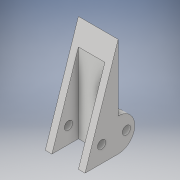
# Autodesk Inventor part: Scooop
Saved by Autodesk Inventor 2019 (Build 230136000, 136)
## iProperties
Created: 2019-05-08
Part Number: Scooop
Material: Generic
Document SubType Name: Modeling
Designer: codubois20
Density: 1 g/cm^3
Appearance: Default
Author: codubois20
Autodesk Inventor part; units mm, degrees
ref_plane "YZ Plane" through (0, 0, 0) normal (1, 0, 0) x (0, 1, 0)
ref_plane "XZ Plane" through (0, 0, 0) normal (0, 1, 0) x (-1, 0, 0)
ref_plane "XY Plane" through (0, 0, 0) normal (0, 0, 1) x (1, 0, 0)
sketch "Sketch1" plane through (0, 0, 0) normal (0, 0, 1) x (1, 0, 0)
  line L0 (0, 0) -> (15.24, 0)
  line L1 (15.24, 0) -> (15.24, 38.1)
  line L2 (15.24, 38.1) -> (0, 38.1)
  line L3 (0, 38.1) -> (0, 0)
  dimension "d4" = 15.24
  dimension "d5" = 38.1
  constraints: 8 end point, 2 parallel, 1 horizontal, 1 perpendicular
  measures "d4" distance of L2.end L1.end
  measures "d5" distance of L1.end L0.end
extrude "Extrusion2" add sketch "Sketch1" along normal blind 12.7
sketch "Sketch8" plane through (0, 0, 12.7) normal (0, 0, 1) x (1, 0, 0)
  line L0 (15.24, 38.1) -> (0, 38.1) projected
  line L1 (0, 38.1) -> (2.54, 38.1)
  line L2 (15.24, 38.1) -> (12.7, 38.1)
  line L3 (0, 0) -> (0, 2.54)
  line L4 (0, 38.1) -> (0, 0) projected
  line L5 (2.54, 2.54) -> (12.7, 2.54)
  line L6 (2.54, 38.1) -> (2.54, 2.54)
  line L7 (12.7, 38.1) -> (12.7, 2.54)
  line L8 (2.54, 38.1) -> (12.7, 38.1)
  line L9 (2.54, 38.1) -> (12.7, 38.1)
  line L10 (2.54, 2.54) -> (12.7, 2.54)
  line L11 (2.54, 38.1) -> (2.54, 2.54)
  line L12 (12.7, 38.1) -> (12.7, 2.54)
  line L13 (2.54, 38.1) -> (12.7, 38.1)
  dimension "d22" = 2.54
  dimension "d23" = 2.54
  dimension "d24" = 2.54
  constraints: 24 end point, 5 perpendicular, 4 collinear, 3 point on line
  measures "d22" distance of L0.end L1.end
  measures "d23" distance of L0.start L2.end
  measures "d24" distance of L3.start L3.end
extrude "Extrusion6" cut sketch "Sketch8" against normal blind 10.16
sketch "Sketch9" plane through (15.24, 0, 0) normal (1, 0, 0) x (0, 0, -1)
  line L0 (-12.7, 2.54) -> (-12.7, 38.1) projected
  line L1 (0, 0) -> (-12.7, 0) projected
  line L2 (0, 38.1) -> (0, 0) projected
  line L3 (0, 38.1) -> (0, 0)
  line L4 (0, 38.1) -> (-12.7, 38.1) projected
  line L5 (0, 38.1) -> (-12.7, 38.1)
  line L6 (0, 38.1) -> (-12.7, 0)
  line L7 (-12.7, 38.1) -> (-12.7, 0) projected
  line L8 (-12.7, 38.1) -> (-12.7, 0)
  constraints: 8 end point, 3 collinear
extrude "Extrusion7" cut sketch "Sketch9" against normal blind 50.8 contours L0 L4 L6 L7
sketch "Sketch10" plane through (0, 0, 0) normal (0, -1, 0) x (1, 0, 0)
  line L0 (12.7, 11.8533) -> (12.7, 2.54) projected
  line L1 (12.7, 11.8533) -> (12.7, 2.54)
  line L2 (12.7, 2.54) -> (2.54, 2.54) projected
  line L3 (12.7, 2.54) -> (2.54, 2.54)
  line L4 (2.54, 2.54) -> (2.54, 12.7)
  line L5 (0, 12.7) -> (15.24, 12.7) projected
  line L6 (12.7, 11.8533) -> (12.7, 12.7)
  line L7 (12.7, 12.7) -> (2.54, 12.7)
  point P0 (0, 0)
  constraints: 10 end point, 3 perpendicular, 2 point on line, 1 collinear
extrude "Extrusion8" cut sketch "Sketch10" against normal blind 2.54
sketch "Sketch11" plane through (15.24, 0, 0) normal (1, 0, 0) x (0, 0, -1)
  line L0 (0, 0) -> (0, 6.35) construction
  line L1 (0, 0) -> (0, 38.1) projected
  line L2 (0, 6.35) -> (6.35, 6.35) construction
  arc A0 (0, 0) -> (6.35, 6.35) centre (0, 6.35) ccw
  arc A1 (6.35, 6.35) -> (0, 12.7) centre (0, 6.35) ccw
  line L3 (0, 12.7) -> (0, 0)
  dimension "d31" = 6.35
  constraints: 6 end point, 5 point on circle, 2 centre point, 2 coincident, 2 point on line, 1 collinear, 1 horizontal
  measures "d31" distance of L0.start L0.end
extrude "Extrusion9" add sketch "Sketch11" against normal blind 3.175
sketch "Sketch12" plane through (15.24, 12.7, 0) normal (1, 0, 0) x (0, 0, -1)
  line L0 (0, 0) -> (0, -12.7) projected
  line L1 (0, -6.35) -> (3.175, -6.35)
  circle A0 centre (3.175, -6.35) radius 1.5875
  dimension "d35" = 3.175
  constraints: 2 end point, 1 centre point, 1 coincident, 1 horizontal, 1 midpoint
  measures "d35" distance of L1.start L1.end
extrude "Extrusion10" cut sketch "Sketch12" against normal blind 3.175
sketch "Sketch13" plane through (15.24, 12.7, 0) normal (1, 0, 0) x (0, 0, -1)
  line L0 (0, -12.7) -> (-12.7, -12.7) projected
  line L1 (-6.35, -12.7) -> (-6.35, -6.35)
  circle A0 centre (-6.35, -6.35) radius 1.5875
  dimension "d38" = 6.35
  dimension "d39" = 3.175
  constraints: 2 end point, 1 centre point, 1 coincident, 1 midpoint, 1 vertical
  measures "d38" distance of L1.start L1.end
  measures "d39" diameter of A0
extrude "Extrusion11" cut sketch "Sketch13" against normal blind 50.8
body "Solid2"
